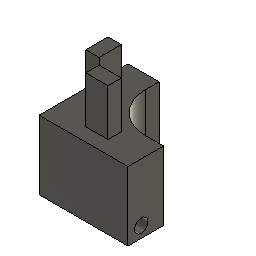
Front Assem (Autodesk Fusion 360 archive; units mm, degrees)
design "Front Base Lower"
Autodesk Fusion 360 part; units mm, degrees
sketch "スケッチ1" plane through (0, 0, 0) normal (0, 0, 1) x (1, 0, 0)
  line L0 (0, 0) -> (20, 0)
  line L1 (20, 0) -> (20, 20)
  line L2 (20, 20) -> (0, 20)
  line L3 (0, 20) -> (0, 0)
  constraint horizontal L0
  constraint vertical L1
  constraint horizontal L2
  constraint vertical L3
  constraint coincident L0.start L3.end
extrude "押し出し1" add sketch "スケッチ1" along normal blind 10.5
sketch "スケッチ2" plane through (0, 0, 10.5) normal (0, 0, 1) x (-1, 0, 0)
  line L0 (0, -20) -> (0, 0)
  line L1 (0, 0) -> (-20, 0)
  line L2 (-20, 0) -> (-20, -20)
  line L3 (-20, -20) -> (0, -20)
  line L4 (-7.5, -3) -> (-12.5, -3)
  line L5 (-12.5, -3) -> (-12.5, -6)
  line L6 (-12.5, -6) -> (-7.5, -6)
  line L7 (-7.5, -6) -> (-7.5, -3)
  line L8 (-6, -12.5) -> (-3, -12.5)
  line L9 (-3, -12.5) -> (-3, -7.5)
  line L10 (-3, -7.5) -> (-6, -7.5)
  line L11 (-6, -7.5) -> (-6, -12.5)
  dimension "d3" = 7.5
  dimension "d4" = 3
  dimension "d5" = 7.5
  dimension "d6" = 3
  constraint horizontal L4
  constraint vertical L5
  constraint horizontal L6
  constraint vertical L7
  constraint horizontal L8
  constraint vertical L9
  constraint horizontal L10
  constraint vertical L11
  measures "d3" distance of L3 L8
  measures "d4" distance of L0 L9
  measures "d5" distance of L0 L7
  measures "d6" distance of L1 L4
extrude "押し出し2" add sketch "スケッチ2" along normal blind 10.5 contours L4 L5 L6 L7 | L8 L9 L10 L11
sketch "スケッチ4" plane through (0, 0, 0) normal (0, 0, -1) x (1, 0, 0)
  line L0 (0, 0) -> (0, -20)
  line L1 (0, -20) -> (20, -20)
  line L2 (20, -20) -> (20, 0)
  line L3 (20, 0) -> (0, 0)
  line L4 (20, -20) -> (7, -20)
  line L5 (7, -20) -> (7, -8)
  line L6 (7, -8) -> (20, -8)
  line L7 (20, -8) -> (20, -20)
  dimension "d14" = 12
  dimension "d15" = 13
  constraint horizontal L4
  constraint vertical L5
  constraint horizontal L6
  constraint vertical L7
  constraint coincident L1.end L2.start
  measures "d14" distance of L1.end L6.end
  measures "d15" distance of L1.end L4.end
extrude "押し出し4" cut sketch "スケッチ4" against normal blind 18 contours L1 L2 L4 L5 L6 L7
fillet "フィレット1" radius 9 1 edges at (7, 8, 5.25)
extrude "押し出し5" add 1 faces at (11.1548, 2.7882, 0) along direction (0, 0, -1) blind 5
sketch "スケッチ3" plane through (20, 0, 0) normal (1, 0, 0) x (0, 1, 0)
  line L0 (8, 10.5) -> (0, 10.5)
  line L1 (0, 10.5) -> (0, -5)
  circle A0 centre (3, -2.5) radius 1.5
  line L2 (8, -5) -> (8, 10.5)
  line L3 (0, -5) -> (8, -5)
  dimension "d9" = 3
  dimension "d10" = 3
  dimension "d22" = 2.5
  measures "d9" diameter of A0
  measures "d10" distance of L1 A0.centre
  measures "d22" distance of A0.centre L3
extrude "押し出し3" cut sketch "スケッチ3" against normal blind 22 contours A0

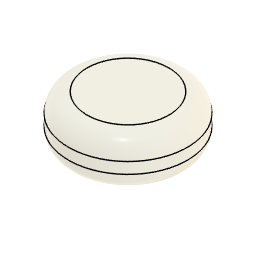
design "Front Wheel"
Autodesk Fusion 360 part; units mm, degrees
sketch "スケッチ1" plane through (0, 0, 0) normal (0, 0, 1) x (1, 0, 0)
  circle A0 centre (0, 0) radius 16
  dimension "d1" = 32
  constraint coincident A0.centre origin
  measures "d1" diameter of A0
extrude "押し出し1" add sketch "スケッチ1" along normal blind 13
fillet "フィレット1" radius 5 2 edges at (-14.9172, -5.7858, 0) (-14.9172, -5.7858, 13)
sketch "スケッチ2" plane through (0, 0, 0) normal (0, 0, -1) x (1, 0, 0)
  circle A0 centre (0, 0) radius 11
  circle A1 centre (0, 0) radius 3
  circle A2 centre (0, 0) radius 1.05
  dimension "d6" = 6
  dimension "d7" = 2.1
  constraint coincident A0.centre A1.centre
  measures "d6" diameter of A1
  measures "d7" diameter of A2
extrude "押し出し2" add sketch "スケッチ2" along normal blind 4 contours A1

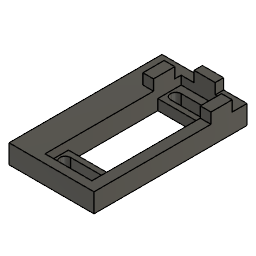
design "サーボモーター土台"
Autodesk Fusion 360 part; units mm, degrees
sketch "スケッチ1" plane through (0, 0, 0) normal (0, 0, 1) x (1, 0, 0)
  line L0 (0, 0) -> (22, 0)
  line L1 (22, 0) -> (22, 42)
  line L2 (22, 42) -> (0, 42)
  line L3 (0, 42) -> (0, 0)
  line L4 (-5, -15) -> (27, -15)
  line L5 (27, -15) -> (27, 57)
  line L6 (27, 57) -> (-5, 57)
  line L7 (-5, 57) -> (-5, -15)
  line L8 (1, 44.5) -> (21, 44.5)
  line L9 (21, 44.5) -> (21, 49.5)
  line L10 (21, 49.5) -> (1, 49.5)
  line L11 (1, 49.5) -> (1, 44.5)
  line L12 (1, 47) -> (21, 47)
  circle A0 centre (3.5, 47) radius 2.5
  circle A1 centre (18.5, 47) radius 2.5
  line L13 (22, 21) -> (-25, 21)
  line L14 (21, -7.5) -> (1, -7.5)
  line L15 (21, -2.5) -> (21, -7.5)
  circle A2 centre (18.5, -5) radius 2.5
  line L16 (1, -2.5) -> (21, -2.5)
  circle A3 centre (3.5, -5) radius 2.5
  line L17 (1, -5) -> (21, -5)
  line L18 (1, -7.5) -> (1, -2.5)
  dimension "d1" = 22
  dimension "d2" = 42
  dimension "d3" = 15
  dimension "d4" = 15
  dimension "d5" = 5
  dimension "d6" = 5
  dimension "d7" = 44.5
  dimension "d8" = 20
  dimension "d9" = 5
  dimension "d10" = 6
  dimension "d11" = 5
  dimension "d12" = 5
  constraint horizontal L0
  constraint vertical L1
  constraint horizontal L2
  constraint vertical L3
  constraint coincident L0.start L3.end
  constraint horizontal L4
  constraint vertical L5
  constraint horizontal L6
  constraint vertical L7
  constraint horizontal L8
  constraint vertical L9
  constraint horizontal L10
  constraint vertical L11
  constraint midpoint L11 L12.start
  constraint midpoint L9 L12.end
  constraint coincident L12 A0.centre
  constraint tangent L11 A0
  constraint coincident L12 A1.centre
  constraint tangent L9 A1
  constraint midpoint L1 L13.start
  constraint perpendicular L7 L13
  constraint symmetric L8.start L13 L16.start
  constraint symmetric L8.end L13 L15.start
  constraint symmetric L9.end L13 L14.start
  constraint symmetric L10.end L13 L14.end
  constraint symmetric L12.start L13 L17.start
  constraint symmetric L12.end L13 L17.end
  constraint symmetric A0 L13 A3
  constraint symmetric A1 L13 A2
  measures "d1" distance of L1.end L2.end
  measures "d2" distance of L0.start L2.end
  measures "d3" distance of L0 L4
  measures "d4" distance of L2 L6
  measures "d5" distance of L1 L5
  measures "d6" distance of L3 L7
  measures "d7" distance of L0 L8
  measures "d8" distance of L9.end L10.end
  measures "d9" distance of L8.end L9.end
  measures "d10" distance of L5 L9
  measures "d11" diameter of A0
  measures "d12" diameter of A1
extrude "押し出し1" add sketch "スケッチ1" along normal blind 5 contours L4 L5 L6 L7 | L8 L11 A0 | L10 L11 A0 | L8 L9 A1 | L9 L10 A1 | L14 L15 A2 | L15 A2 L16 | L14 A3 L18 | L16 A3 L18
sketch "スケッチ2" plane through (0, 0, 5) normal (0, 0, 1) x (-1, 0, 0)
  line L0 (0, 0) -> (0, -42)
  line L1 (0, -42) -> (-22, -42)
  line L2 (-22, -42) -> (-22, 0)
  line L3 (-22, 0) -> (0, 0)
  arc A0 (-18.5, -44.5) -> (-18.5, -49.5) centre (-18.5, -47) ccw
  line L4 (-18.5, -44.5) -> (-3.5, -44.5)
  arc A1 (-3.5, -49.5) -> (-3.5, -44.5) centre (-3.5, -47) ccw
  line L5 (-3.5, -49.5) -> (-18.5, -49.5)
  line L6 (5, -57) -> (5, 15)
  line L7 (5, 15) -> (-27, 15)
  line L8 (-27, 15) -> (-27, -57)
  line L9 (-27, -57) -> (5, -57)
  line L10 (5, -57) -> (-27, -57)
  line L11 (-27, -57) -> (-27, 15)
  line L12 (-27, 15) -> (5, 15)
  line L13 (5, 15) -> (5, -57)
  line L14 (0, -42) -> (-22, -42)
  line L15 (-22, -42) -> (-22, -53)
  line L16 (-22, -53) -> (0, -53)
  line L17 (0, -53) -> (0, -42)
  arc A2 (-18.5, 7.5) -> (-18.5, 2.5) centre (-18.5, 5) ccw
  line L18 (-18.5, 7.5) -> (-3.5, 7.5)
  arc A3 (-3.5, 2.5) -> (-3.5, 7.5) centre (-3.5, 5) ccw
  line L19 (-3.5, 2.5) -> (-18.5, 2.5)
  line L20 (-22, -21) -> (22.5657, -21)
  arc A4 (-3.5, 2.5) -> (-3.5, 7.5) centre (-3.5, 5) ccw
  line L21 (-18.5, 2.5) -> (-3.5, 2.5)
  line L22 (0, 0) -> (-22, 0)
  line L23 (0, 11) -> (0, 0)
  line L24 (-3.5, 7.5) -> (-18.5, 7.5)
  arc A5 (-18.5, 7.5) -> (-18.5, 2.5) centre (-18.5, 5) ccw
  line L25 (-22, 11) -> (0, 11)
  line L26 (-22, 0) -> (-22, 11)
  line L27 (0, 0) -> (-22, 0)
  constraint horizontal L10
  constraint vertical L11
  constraint horizontal L12
  constraint vertical L13
  constraint coincident L7.end L8.start
  constraint coincident L6.start L9.end
  constraint horizontal L14
  constraint vertical L15
  constraint horizontal L16
  constraint vertical L17
  constraint coincident L0.end L1.start
  constraint midpoint L2 L20.start
  constraint perpendicular L2 L20
  constraint symmetric L0.end L20 L0.start
  constraint symmetric L1.end L20 L2.end
  constraint symmetric A0.start L20 A2.end
  constraint symmetric A0.end L20 A2.start
  constraint symmetric A0 L20 A5
  constraint symmetric L4.end L20 A3.start
  constraint symmetric A1.start L20 L18.end
  constraint symmetric A1 L20 A4
  constraint symmetric L15.end L20 L25.start
  constraint symmetric L16.end L20 L23.start
extrude "押し出し2" add sketch "スケッチ2" along normal blind 4 contours L6 L7 L8 L9 L10 L11 L12 L13
sketch "スケッチ3" plane through (0, 0, 9) normal (0, 0, 1) x (-1, 0, 0)
  line L0 (-22, -53) -> (-22, 11)
  line L1 (0, 11) -> (0, -53)
  line L2 (0, -53) -> (-22, -53)
  line L3 (5, 15) -> (-27, 15)
  line L4 (-27, 15) -> (-27, -57)
  line L5 (-27, -57) -> (5, -57)
  line L6 (5, -57) -> (5, 15)
  line L7 (-16, -53) -> (-6, -53)
  line L8 (-6, -53) -> (-6, -57)
  line L9 (-6, -57) -> (-16, -57)
  line L10 (-16, -57) -> (-16, -53)
  line L11 (-22, 11) -> (0, 11)
  line L12 (-22, -50) -> (-27, -50)
  line L13 (-27, -50) -> (-27, -40)
  line L14 (-27, -40) -> (-22, -40)
  line L15 (-22, -40) -> (-22, -50)
  line L16 (0, -40) -> (5, -40)
  line L17 (5, -40) -> (5, -50)
  line L18 (5, -50) -> (0, -50)
  line L19 (0, -50) -> (0, -40)
  dimension "d17" = 11
  constraint horizontal L7
  constraint vertical L8
  constraint horizontal L9
  constraint vertical L10
  constraint coincident L5 L8.end
  constraint coincident L2 L7.start
  constraint horizontal L12
  constraint vertical L13
  constraint horizontal L14
  constraint vertical L15
  constraint coincident L4 L13.end
  constraint coincident L0 L12.start
  constraint horizontal L16
  constraint vertical L17
  constraint horizontal L18
  constraint vertical L19
  constraint coincident L1 L16.start
  measures "d17" distance of L4 L10
extrude "押し出し3" add sketch "スケッチ3" along normal blind 5 contours L0 L4 L12 L13 L14 L15 | L2 L5 L7 L8 L9 L10 | L1 L6 L16 L17 L18 L19
sketch "スケッチ5" plane through (-5, 0, 0) normal (-1, 0, 0) x (0, -1, 0)
  line L0 (-57, 0) -> (15, 0)
  line L1 (15, 0) -> (15, 9)
  line L2 (15, 9) -> (-40, 9)
  line L3 (-40, 9) -> (-40, 14)
  line L4 (-40, 14) -> (-50, 14)
  line L5 (-50, 14) -> (-50, 9)
  line L6 (-50, 9) -> (-57, 9)
  line L7 (-57, 9) -> (-57, 0)
  line L8 (15, 0) -> (-57, 0)
  line L9 (-57, 0) -> (-57, 9)
  line L10 (-57, 9) -> (15, 9)
  line L11 (15, 9) -> (15, 0)
  constraint horizontal L8
  constraint vertical L9
  constraint horizontal L10
  constraint vertical L11
  constraint coincident L6.end L7.start
  constraint coincident L0.end L1.start
extrude "押し出し5" add sketch "スケッチ5" along normal blind 8 contours L0 L1 L2 L6 L7 L8 L9 L10 L11

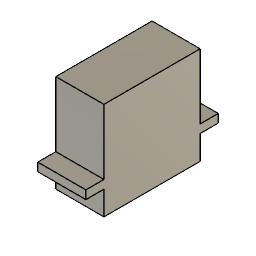
design "サーボモータ模型"
Autodesk Fusion 360 part; units mm, degrees
sketch "スケッチ1" plane through (0, 0, 0) normal (0, 0, 1) x (1, 0, 0)
  line L0 (0, 0) -> (20, 0)
  line L1 (20, 0) -> (20, 40)
  line L2 (20, 40) -> (0, 40)
  line L3 (0, 40) -> (0, 0)
  dimension "d1" = 20
  dimension "d2" = 40
  constraint horizontal L0
  constraint vertical L1
  constraint horizontal L2
  constraint vertical L3
  constraint coincident L0.start L3.end
  measures "d1" distance of L1.end L2.end
  measures "d2" distance of L0.start L2.end
extrude "押し出し1" add sketch "スケッチ1" along normal blind 10
sketch "スケッチ2" plane through (0, 0, 10) normal (0, 0, 1) x (-1, 0, 0)
  line L0 (0, -40) -> (0, 0)
  line L1 (0, 0) -> (-20, 0)
  line L2 (-20, 0) -> (-20, -40)
  line L3 (-20, -40) -> (0, -40)
  line L4 (0, -47.5) -> (-20, -47.5)
  line L5 (-20, -47.5) -> (-20, 7.5)
  line L6 (-20, 7.5) -> (0, 7.5)
  line L7 (0, 7.5) -> (0, -47.5)
  dimension "d5" = 55
  dimension "d6" = 7.5
  constraint horizontal L4
  constraint vertical L5
  constraint horizontal L6
  constraint vertical L7
  measures "d5" distance of L4.start L6.end
  measures "d6" distance of L3 L4
extrude "押し出し2" add sketch "スケッチ2" along normal blind 3.5
sketch "スケッチ3" plane through (0, 0, 13.5) normal (0, 0, 1) x (-1, 0, 0)
  line L0 (0, 7.5) -> (-20, 7.5)
  line L1 (-20, 7.5) -> (-20, -47.5)
  line L2 (-20, -47.5) -> (0, -47.5)
  line L3 (0, -47.5) -> (0, 7.5)
  line L4 (0, 0) -> (-20, 0)
  line L5 (-20, 0) -> (-20, -40)
  line L6 (-20, -40) -> (0, -40)
  line L7 (0, -40) -> (0, 0)
  dimension "d9" = 40
  constraint horizontal L4
  constraint vertical L5
  constraint horizontal L6
  constraint vertical L7
  constraint coincident L1 L5.end
  constraint coincident L4.start L7.end
  measures "d9" distance of L4.end L5.end
extrude "押し出し3" add sketch "スケッチ3" along normal blind 27 contours L1 L3 L4 L5 L6 L7
sketch "スケッチ4" plane through (0, 0, 0) normal (0, 0, -1) x (1, 0, 0)
  line L0 (0, 0) -> (0, -40)
  line L1 (0, -40) -> (20, -40)
  line L2 (20, -40) -> (20, 0)
  line L3 (20, 0) -> (0, 0)
  circle A0 centre (10, -10) radius 3
  dimension "d12" = 6
  measures "d12" diameter of A0
extrude "押し出し4" add sketch "スケッチ4" along normal blind 6.5 contours A0

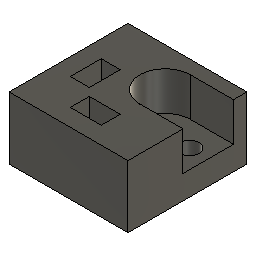
design "Front Base Upper"
Autodesk Fusion 360 part; units mm, degrees
sketch "スケッチ1" plane through (0, 0, 0) normal (0, 0, 1) x (1, 0, 0)
  line L0 (0, 0) -> (20, 0)
  line L1 (20, 0) -> (20, 20)
  line L2 (20, 20) -> (0, 20)
  line L3 (0, 20) -> (0, 0)
  dimension "d1" = 20
  dimension "d2" = 20
  constraint horizontal L0
  constraint vertical L1
  constraint horizontal L2
  constraint vertical L3
  constraint coincident L0.start L3.end
  measures "d1" distance of L1.end L2.end
  measures "d2" distance of L0.start L2.end
extrude "押し出し1" add sketch "スケッチ1" along normal blind 21
sketch "スケッチ2" plane through (20, 0, 0) normal (1, 0, 0) x (0, 1, 0)
  line L0 (0, 0) -> (20, 0)
  line L1 (20, 0) -> (20, 21)
  line L2 (20, 21) -> (0, 21)
  line L3 (0, 21) -> (0, 0)
  circle A0 centre (5, 5) radius 1.15
  dimension "d5" = 2.3
  dimension "d8" = 5
  dimension "d11" = 5
  measures "d5" diameter of A0
  measures "d8" distance of L3 A0.centre
  measures "d11" distance of L0 A0.centre
extrude "押し出し2" cut sketch "スケッチ2" against normal blind 25 contours A0
sketch "スケッチ7" plane through (0, 0, 21) normal (0, 0, 1) x (-1, 0, 0)
  line L0 (0, -20) -> (0, 0)
  line L1 (0, 0) -> (-20, 0)
  line L2 (-20, 0) -> (-20, -20)
  line L3 (-20, -20) -> (0, -20)
  line L4 (-12.75, -17.75) -> (-20, -17.75)
  line L5 (-20, -17.75) -> (-20, -9.25)
  line L6 (-20, -9.25) -> (-12.75, -9.25)
  line L7 (-8.5, -13.5) -> (-20, -13.5)
  circle A0 centre (-12.85, -13.5) radius 1.6
  circle A1 centre (-16.85, -13.5) radius 1.6
  arc A2 (-12.75, -17.75) -> (-8.5, -13.5) centre (-12.75, -13.5) ccw
  arc A3 (-8.5, -13.5) -> (-12.75, -9.25) centre (-12.75, -13.5) ccw
  point P0 (-8.5, -17.75)
  point P1 (-8.5, -9.25)
  dimension "d16" = 8.5
  dimension "d17" = 11.5
  dimension "d18" = 3.2
  dimension "d19" = 3.2
  dimension "d20" = 4
  dimension "d21" = 4.35
  dimension "d22" = 4.25
  dimension "d23" = 4.25
  dimension "d24" = 4.25
  constraint horizontal L4
  constraint vertical L5
  constraint horizontal L6
  constraint coincident L2 L5.end
  constraint coincident L5 L7.end
  constraint perpendicular L5 L7
  constraint coincident L7 A0.centre
  constraint coincident L7 A1.centre
  constraint coincident P0 L4
  constraint tangent L4 A2
  constraint coincident P1 L6
  constraint tangent L6 A3
  constraint coincident L7.start A2.end
  measures "d16" distance of P0 P1
  measures "d17" distance of P0 L4.end
  measures "d18" diameter of A0
  measures "d19" diameter of A1
  measures "d20" distance of A0.centre A1.centre
  measures "d21" distance of L7.start A0.centre
  measures "d22" radius of A2
  measures "d23" distance of L4 L7
  measures "d24" radius of A3
extrude "押し出し4" cut sketch "スケッチ7" against normal blind 6.5 contours L2 L4 L5 L7 A0 A1 A2 | L2 L5 L6 L7 A0 A1 A3
extrude "押し出し5" cut 2 faces at (12.2215, 13.3267, 21) (16.1057, 13.3074, 21) along direction (0, 0, -1) blind 26
sketch "スケッチ11" plane through (20, 0, 0) normal (1, 0, 0) x (0, 1, 0)
  line L0 (17.75, 21) -> (17.75, 14.5)
  line L1 (17.75, 14.5) -> (9.25, 14.5)
  line L2 (9.25, 14.5) -> (9.25, 21)
  line L3 (9.25, 21) -> (0, 21)
  line L4 (0, 21) -> (0, 0)
  line L5 (0, 0) -> (20, 0)
  line L6 (20, 0) -> (20, 21)
  line L7 (20, 21) -> (17.75, 21)
  circle A0 centre (5, 5) radius 1.15
  line L8 (0, 10.5) -> (20, 10.5)
  line L9 (20, 10.5) -> (20, 0)
  line L10 (20, 0) -> (0, 0)
  line L11 (0, 0) -> (0, 10.5)
  dimension "d34" = 4
  constraint horizontal L8
  constraint vertical L9
  constraint horizontal L10
  constraint vertical L11
  constraint coincident L5.end L6.start
  constraint coincident L4 L8.start
  measures "d34" distance of L1 L8
extrude "押し出し8" cut sketch "スケッチ11" against normal blind 32 contours L4 L5 L6 L8 L9 L10 L11
sketch "スケッチ12" plane through (0, 0, 21) normal (0, 0, 1) x (-1, 0, 0)
  line L0 (-12.75, -17.75) -> (-20, -17.75)
  line L1 (-20, -17.75) -> (-20, -20)
  line L2 (-20, -20) -> (0, -20)
  line L3 (0, -20) -> (0, 0)
  line L4 (0, 0) -> (-20, 0)
  line L5 (-20, 0) -> (-20, -9.25)
  line L6 (-20, -9.25) -> (-12.75, -9.25)
  arc A0 (-12.75, -17.75) -> (-12.75, -9.25) centre (-12.75, -13.5) ccw
  line L7 (-2.9, -12.6) -> (-6.1, -12.6)
  line L8 (-6.1, -12.6) -> (-6.1, -7.4)
  line L9 (-6.1, -7.4) -> (-2.9, -7.4)
  line L10 (-2.9, -7.4) -> (-2.9, -12.6)
  line L11 (-12.6, -2.9) -> (-7.4, -2.9)
  line L12 (-7.4, -2.9) -> (-7.4, -6.1)
  line L13 (-7.4, -6.1) -> (-12.6, -6.1)
  line L14 (-12.6, -6.1) -> (-12.6, -2.9)
  dimension "d37" = 2.9
  dimension "d38" = 5.2
  dimension "d39" = 3.2
  dimension "d40" = 7.4
  dimension "d41" = 3.2
  dimension "d42" = 5.2
  dimension "d43" = 2.9
  dimension "d44" = 7.4
  constraint horizontal L7
  constraint vertical L8
  constraint horizontal L9
  constraint vertical L10
  constraint horizontal L11
  constraint vertical L12
  constraint horizontal L13
  constraint vertical L14
  measures "d37" distance of L4 L11
  measures "d38" distance of L12.end L13.end
  measures "d39" distance of L11.start L13.end
  measures "d40" distance of L5 L14
  measures "d41" distance of L7.start L7.end
  measures "d42" distance of L7.end L8.end
  measures "d43" distance of L3 L10
  measures "d44" distance of L2 L7
extrude "押し出し9" cut sketch "スケッチ12" against normal blind 22 contours L7 L8 L9 L10 | L11 L12 L13 L14
equation "d40 = 10 mm - 2.6 mm"

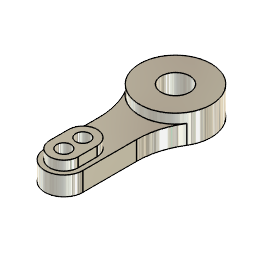
design "サーボハンドル"
Autodesk Fusion 360 part; units mm, degrees
sketch "スケッチ1" plane through (0, 0, 0) normal (0, 0, 1) x (1, 0, 0)
  line L0 (0, 0) -> (15, 0)
  line L1 (15, 0) -> (15, 35)
  line L2 (15, 35) -> (0, 35)
  line L3 (0, 35) -> (0, 0)
  circle A0 centre (7.5, 27.5) radius 7.5
  line L4 (3.5, 0) -> (11.5, 0)
  line L5 (11.5, 0) -> (11.5, 21.1557)
  line L6 (11.5, 21.1557) -> (3.5, 21.1557)
  line L7 (3.5, 21.1557) -> (3.5, 0)
  dimension "d1" = 8
  dimension "d2" = 3.5
  dimension "d4" = 35
  dimension "d5" = 15
  constraint horizontal L0
  constraint vertical L1
  constraint horizontal L2
  constraint vertical L3
  constraint coincident L0.start L3.end
  constraint tangent L3 A0
  constraint tangent L2 A0
  constraint horizontal L4
  constraint vertical L5
  constraint horizontal L6
  constraint vertical L7
  constraint coincident L0 L4.start
  constraint coincident A0 L6.end
  measures "d1" distance of L5.end L6.end
  measures "d2" distance of L3 L7
  measures "d4" distance of L2 L4
  measures "d5" diameter of A0
extrude "押し出し1" add sketch "スケッチ1" along normal blind 6 contours L0 A0 L4 L5 L7 | A0 L6 | A0 L6
fillet "フィレット1" radius 15.5 2 edges at (3.5, 21.1557, 3) (11.5, 21.1557, 3)
fillet "フィレット1" radius 4 2 edges at (3.5, 0, 3) (11.5, 0, 3)
sketch "スケッチ2" plane through (0, 0, 6) normal (0, 0, 1) x (-1, 0, 0)
  arc A0 (-3.5, -4) -> (-11.5, -4) centre (-7.5, -4) ccw
  line L0 (-11.5, -4) -> (-11.5, -15.3037)
  arc A1 (-13.8587, -23.5229) -> (-11.5, -15.3037) centre (-27, -15.3037) ccw
  arc A2 (-13.8587, -23.5229) -> (-1.1413, -23.5229) centre (-7.5, -27.5) ccw
  arc A3 (-3.5, -15.3037) -> (-1.1413, -23.5229) centre (12, -15.3037) ccw
  line L1 (-3.5, -15.3037) -> (-3.5, -4)
  line L2 (-10.5, -4) -> (-10.5, -8)
  line L3 (-4.5, -8) -> (-4.5, -4)
  arc A4 (-4.5, -4) -> (-7.5, -1) centre (-7.5, -4) ccw
  arc A5 (-7.5, -1) -> (-10.5, -4) centre (-7.5, -4) ccw
  arc A6 (-7.5, -11) -> (-4.5, -8) centre (-7.5, -8) ccw
  arc A7 (-10.5, -8) -> (-7.5, -11) centre (-7.5, -8) ccw
  circle A8 centre (-7.5, -27.5) radius 7.5
  point P0 (-4.5, -1)
  point P1 (-10.5, -1)
  point P2 (-4.5, -11)
  dimension "d12" = 6
  dimension "d13" = 10
  dimension "d14" = 1
  dimension "d16" = 3
  constraint vertical L2
  constraint vertical L3
  constraint coincident P0 L3
  constraint tangent L3 A4
  constraint coincident P1 L2
  constraint tangent L2 A5
  constraint equal A4 A5
  constraint coincident A4.end A5.start
  constraint coincident P2 L3
  constraint tangent L3 A6
  constraint equal A4 A6
  constraint tangent L2 A7
  constraint equal A4 A7
  constraint coincident A6.start A7.end
  measures "d12" distance of P0 P1
  measures "d13" distance of P0 P2
  measures "d14" distance of L1 L3
  measures "d16" radius of A4
extrude "押し出し2" cut sketch "スケッチ2" against normal blind 2 contours A0 L0 A1 A3 L1 A8
sketch "スケッチ3" plane through (0, 0, 6) normal (0, 0, 1) x (-1, 0, 0)
  line L0 (-10.5, -4) -> (-10.5, -8)
  arc A0 (-10.5, -8) -> (-4.5, -8) centre (-7.5, -8) ccw
  line L1 (-4.5, -8) -> (-4.5, -4)
  arc A1 (-4.5, -4) -> (-10.5, -4) centre (-7.5, -4) ccw
  circle A2 centre (-7.5, -8) radius 1.5
  circle A3 centre (-7.5, -4) radius 1.5
  line L2 (-7.5, -8) -> (-7.5, -4)
  line L3 (-4, 0) -> (-13, 0)
  arc A4 (-3.5, -4) -> (-11.5, -4) centre (-7.5, -4) ccw
  circle A5 centre (-7.5, -27.5) radius 3
  circle A6 centre (-7.5, -27.5) radius 7.5
  dimension "d20" = 4
  dimension "d21" = 3
  dimension "d22" = 3
  dimension "d23" = 3
  dimension "d24" = 4
  dimension "d27" = 6
  constraint coincident A0.centre A2.centre
  constraint coincident A1.centre A3.centre
  constraint parallel L1 L2
  constraint horizontal L3
  constraint tangent L3 A4
  constraint concentric A5 A6
  measures "d20" distance of A0.centre A1.centre
  measures "d21" diameter of A2
  measures "d22" diameter of A3
  measures "d23" distance of L1 L2
  measures "d24" distance of A1.centre L3
  measures "d27" diameter of A5
extrude "押し出し3" cut sketch "スケッチ3" against normal blind 6 contours A2 | A3 | A5
